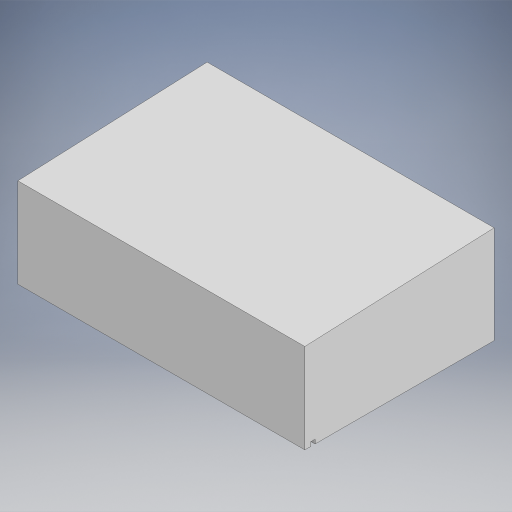
# Autodesk Inventor part: Part2
Saved by Autodesk Inventor 2023.1 (Build 271208000, 208)
## iProperties
RuleStatus: InUse
Created: 2022-10-28
Part Number: Part2
Material: Generic
Document SubType Name: Modeling
Designer: awelt
Mass: 19287.9 g
Surface Area: 4871.17 cm^2
Volume: 19287.9 cm^3
Density: 1 g/cm^3
Appearance: Default
AfterAnyParamChange0: BoundingBox
AfterAnyiPropertyChange0: BoundingBox
PartBodyChanged0: BoundingBox
BoundingBL1: 6
BoundingBL2: 11 5/8
BoundingBL3: 17 5/8
BoundingCF: 0.711
Author: awelt
Autodesk Inventor part; units mm, degrees
ref_plane "YZ Plane" through (0, 0, 0) normal (1, 0, 0) x (0, 1, 0)
ref_plane "XZ Plane" through (0, 0, 0) normal (0, 1, 0) x (-1, 0, 0)
ref_plane "XY Plane" through (0, 0, 0) normal (0, 0, 1) x (1, 0, 0)
sketch "Sketch2" plane through (0, 0, 0) normal (1, 0, 0) x (0, 1, 0)
  line L0 (0, 0) -> (152.4, 0)
  line L1 (152.4, 0) -> (152.4, -295.275)
  line L2 (152.4, -295.275) -> (0, -295.275)
  line L3 (0, -295.275) -> (0, 0)
  line L4 (152.4, -295.275) -> (139.7, 0)
  line L5 (0, -9.525) -> (6.35, -9.525)
  line L6 (6.35, -9.525) -> (6.35, -15.875)
  line L7 (6.35, -15.875) -> (0, -15.875)
  line L8 (0, -15.875) -> (0, -9.525)
  point P0 (0, -15.875)
  dimension "d4" = 152.4
  dimension "d5" = 295.275
  dimension "d6" = 12.7
  dimension "d7" = 6.35
  dimension "d8" = 6.35
  dimension "d9" = 9.525
  constraints: 18 end point, 4 parallel, 2 horizontal, 2 perpendicular, 2 point on line
  measures "d4" distance of L1.end L2.end
  measures "d5" distance of L0.end L1.end
  measures "d6" distance of L4.end L0.end
  measures "d7" distance of L6.end L7.end
  measures "d8" distance of L5.end L6.end
  measures "d9" distance of L5.start L0.start
extrude "Extrusion2" add sketch "Sketch2" along normal blind 447.675 contours L0 L4 L2 L3 L7 L6 L5
body "Solid2"
